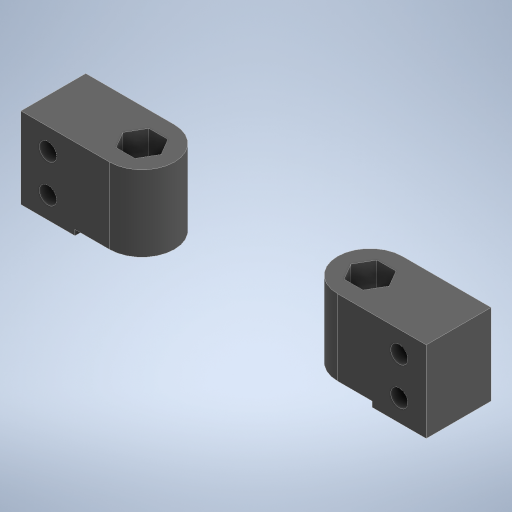
# Autodesk Inventor part: wheel_setter
Saved by Autodesk Inventor 2024.1 (Build 281209000, 209)
## iProperties
Created: 2025-01-09
Part Number: wheel_setter
Material: 一般
Document SubType Name: Modeling
Designer: hibik
Density: 1 g/cm^3
Appearance: 既定
Author: hibik
Autodesk Inventor part; units mm, degrees
ref_plane "YZ Plane" through (0, 0, 0) normal (1, 0, 0) x (0, 1, 0)
ref_plane "XZ Plane" through (0, 0, 0) normal (0, 1, 0) x (-1, 0, 0)
sketch "スケッチ1" plane through (0, 0, 0) normal (0, 1, 0) x (-1, 0, 0)
  line L0 (-3.5218, 0) -> (-1.7609, 3.05)
  line L1 (-1.7609, 3.05) -> (1.7609, 3.05)
  line L2 (1.7609, 3.05) -> (3.5218, 0)
  line L3 (3.5218, 0) -> (1.7609, -3.05)
  line L4 (1.7609, -3.05) -> (-1.7609, -3.05)
  line L5 (-1.7609, -3.05) -> (-3.5218, 0)
  circle A0 centre (0, 0) radius 6
  line L6 (0, 6) -> (16.4, 6)
  line L7 (16.4, 6) -> (16.4, -6)
  line L8 (16.4, -6) -> (0, -6)
  line L9 (0, -6) -> (0, 6)
  point P0 (0, -6)
  dimension "d1" = 12
  dimension "d0" = 6.1
  dimension "d2" = 16.4
  constraints: 20 end point, 4 horizontal, 2 coincident, 2 parallel, 1 perpendicular, 16 other
  measures "d0" distance between parallel lines of L4 L1
  measures "d2" distance of L6.start L6.end
extrude "押し出し1" add sketch "スケッチ1" along normal blind 12 contours L5 L4 L9 A0 L1 L0 | L9 A0 L4 L3 L2 L1 | L6 L7 L8 A0
sketch "スケッチ2" plane through (0, 0, -6) normal (0, 0, -1) x (-1, 0, 0)
  line L0 (0, 12) -> (16.4, 12) projected
  line L1 (16.4, 12) -> (6.4, 12)
  line L2 (6.4, 12) -> (6.4, -3)
  line L3 (6.4, -3) -> (16.4, -3)
  line L4 (16.4, -3) -> (16.4, 12)
  point P0 (0, 0)
  dimension "d5" = 10
  dimension "d6" = 15
  constraints: 8 end point, 2 parallel, 1 horizontal, 1 perpendicular
  measures "d5" distance of L3.end L2.end
  measures "d6" distance of L2.end L1.end
extrude "押し出し2" add sketch "スケッチ2" against normal up to surface (12 mm away)
sketch "スケッチ3" plane through (0, 12, -6) normal (0, 0, -1) x (-1, 0, 0)
  line L0 (14.6909, -4) -> (13.0454, -6.85)
  line L1 (13.0454, -6.85) -> (9.7546, -6.85)
  line L2 (9.7546, -6.85) -> (8.1091, -4)
  line L3 (8.1091, -4) -> (9.7546, -1.15)
  line L4 (9.7546, -1.15) -> (13.0454, -1.15)
  line L5 (13.0454, -1.15) -> (14.6909, -4)
  line L6 (9.7546, -13.85) -> (8.1091, -11)
  line L7 (8.1091, -11) -> (9.7546, -8.15)
  line L8 (9.7546, -8.15) -> (13.0454, -8.15)
  line L9 (13.0454, -8.15) -> (14.6909, -11)
  line L10 (14.6909, -11) -> (13.0454, -13.85)
  line L11 (13.0454, -13.85) -> (9.7546, -13.85)
  line L12 (16.4, -15) -> (16.4, 0) projected
  line L13 (16.4, -7.5) -> (20.3002, -7.5)
  circle A0 centre (11.4, -4) radius 1.6
  circle A1 centre (11.4, -11) radius 1.6
  point P0 (0, -12)
  dimension "d9" = 5.7
  dimension "d10" = 3.5
  dimension "d11" = 5
  dimension "d14" = 3.2
  dimension "d15" = 3.2
  constraints: 26 end point, 3 horizontal, 2 centre point, 2 coincident, 1 midpoint, 1 parallel, 1 symmetric about line, 1 vertical alignment, 26 other
  measures "d9" distance between parallel lines of L1 L4
  measures "d10" distance from line of point (11.4, -11) L13
  measures "d11" distance from line of L12 point (11.4, -4)
  measures "d14" diameter of A0
  measures "d15" diameter of A1
extrude "押し出し3" cut sketch "スケッチ3" against normal blind 3 contours L0 L1 L2 L3 L4 L5 | L6 L7 L8 L9 L10 L11 | A0 | A1
extrude "押し出し4" cut sketch "スケッチ3" against normal through all contours A0 | A1
ref_plane "作業平面1" through (21.1, 12, -6) normal (-1, 0, 0) x (0, 0, 1)
sketch "スケッチ4" plane through (0, 0, 0) normal (0, -1, 0) x (1, 0, 0)
  circle A0 centre (0, 0) radius 5.3
  line L0 (1.7609, 3.05) -> (-1.7609, 3.05) projected
  line L1 (3.5218, 0) -> (1.7609, 3.05) projected
  line L2 (1.7609, -3.05) -> (3.5218, 0) projected
  line L3 (-1.7609, -3.05) -> (1.7609, -3.05) projected
  line L4 (-3.5218, 0) -> (-1.7609, -3.05) projected
  line L5 (-1.7609, 3.05) -> (-3.5218, 0) projected
  line L6 (-6.4, 6) -> (-6.4, -6) projected
  line L7 (0, -6) -> (-6.4, -6) projected
  arc A1 (0, -6) -> (0, 6) centre (0, 0) ccw projected
  line L8 (-6.4, 6) -> (0, 6) projected
  dimension "d19" = 10.6
  constraints: 1 centre point, 1 coincident
  measures "d19" diameter of A0
extrude "押し出し5" add sketch "スケッチ4" along normal blind 2 contours L8 A1 L7 L6
mirror "ミラー2" about plane through (21.1, 12, -6) normal (-1, 0, 0)
